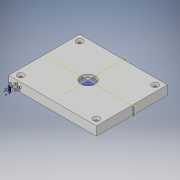
# Autodesk Inventor part: Masterboxtop
Saved by Autodesk Inventor 2019 (Build 230136000, 136)
## iProperties
Created: 2019-08-02
Part Number: Masterboxtop
Material: Generic
Document SubType Name: Modeling
Designer: Riley
Density: 1 g/cm^3
Appearance: Default
Author: Riley
Autodesk Inventor part; units mm, degrees
ref_plane "YZ Plane" through (0, 0, 0) normal (1, 0, 0) x (0, 1, 0)
ref_plane "XZ Plane" through (0, 0, 0) normal (0, 1, 0) x (-1, 0, 0)
ref_plane "XY Plane" through (0, 0, 0) normal (0, 0, 1) x (1, 0, 0)
sketch "Sketch1" plane through (0, 0, 0) normal (0, 1, 0) x (-1, 0, 0)
  line L0 (0, 0) -> (89.789, 0)
  line L1 (89.789, 0) -> (89.789, 71.3232)
  line L2 (89.789, 71.3232) -> (0, 71.3232)
  line L3 (0, 71.3232) -> (0, 0)
  line L4 (93.345, 74.8792) -> (-3.556, 74.8792)
  line L5 (-3.556, 74.8792) -> (-3.556, -3.556)
  line L6 (-3.556, -3.556) -> (93.345, -3.556)
  line L7 (93.345, -3.556) -> (93.345, 74.8792)
  dimension "d0" = 89.789
  dimension "d1" = 71.3232
  dimension "d2" = 3.556
  dimension "d3" = 3.556
  dimension "d4" = 3.556
  dimension "d5" = 3.556
  constraints: 16 end point, 4 parallel, 2 horizontal, 2 perpendicular
  measures "d0" distance of L2.end L1.end
  measures "d1" distance of L1.end L0.end
  measures "d2" distance between parallel lines of L4 L2
  measures "d3" distance between parallel lines of L7 L1
  measures "d4" distance between parallel lines of L6 L0
  measures "d5" distance between parallel lines of L5 L3
extrude "Extrusion1" add sketch "Sketch1" along normal blind 6.35
sketch "Sketch2" plane through (0, 6.35, 0) normal (0, 1, 0) x (1, 0, 0)
  line L0 (-93.345, 3.556) -> (3.556, 3.556)
  line L1 (3.556, 3.556) -> (3.556, -74.8792)
  line L2 (3.556, -74.8792) -> (-93.345, -74.8792)
  line L3 (-93.345, -74.8792) -> (-93.345, 3.556)
  point P0 (0, 0)
  dimension "d8" = 78.4352
  dimension "d9" = 96.901
  constraints: 8 end point, 2 parallel, 1 horizontal, 1 perpendicular
  measures "d8" distance between parallel lines of L2 L0
  measures "d9" distance between parallel lines of L1 L3
extrude "Extrusion2" add sketch "Sketch2" along normal blind 3.556
sketch "Sketch3" plane through (0, 9.906, 0) normal (0, 1, 0) x (1, 0, 0)
  circle A0 centre (-44.8945, -35.6616) radius 7.9883
  line L0 (-93.345, 3.556) -> (-93.345, -74.8792) projected
  line L1 (3.556, 3.556) -> (-93.345, 3.556) projected
  point P0 (0, 0)
  dimension "d12" = 48.4505
  dimension "d13" = 39.2176
  dimension "d14" = 15.9766
  constraints: 1 centre point
  measures "d12" distance from line of L0 A0.centre
  measures "d13" distance from line of L1 A0.centre
  measures "d14" diameter of A0
extrude "Extrusion3" cut sketch "Sketch3" against normal blind 3.556 and the other way blind 1.016
sketch "Sketch5" plane through (-93.345, 0, -3.556) normal (-1, 0, 0) x (0, 0, 1)
  line L0 (78.4352, 0) -> (0, 0) projected
  line L1 (78.4352, 0) -> (77.1652, 0)
  line L2 (77.1652, 0) -> (77.1652, -7.62)
  line L3 (77.1652, -7.62) -> (78.4352, -7.62)
  line L4 (78.4352, -7.62) -> (78.4352, 0)
  line L5 (77.1652, -7.62) -> (76.4032, -6.5318)
  line L6 (76.4032, -6.5318) -> (76.4032, -2.54)
  line L7 (76.4032, -2.54) -> (77.1652, -2.54)
  point P0 (3.556, 0)
  dimension "d19" = 1.27
  dimension "d20" = 7.62
  dimension "d21" = 35
  dimension "d22" = 5.08
  dimension "d23" = 0.762
  constraints: 14 end point, 2 parallel, 2 perpendicular, 1 horizontal, 1 point on line, 1 vertical
  measures "d19" distance between parallel lines of L2 L4
  measures "d20" distance between parallel lines of L0 L3
  measures "d21" angle of L5 L2
  measures "d22" distance between parallel lines of L3 L7
  measures "d23" distance between parallel lines of L2 L6
sketch "Sketch7" plane through (0, 9.906, 0) normal (0, 1, 0) x (1, 0, 0)
  circle A0 centre (-3.1305, -3.1305) radius 1.3525
  line L0 (0, 0) -> (0, -71.3232) projected
  line L1 (-89.789, 0) -> (0, 0) projected
  circle A1 centre (-3.1305, -3.1305) radius 3.1306
  dimension "d40" = 2.7051
  dimension "d41" = 6.2611
  constraints: 2 centre point, 2 tangent, 1 coincident
  measures "d40" diameter of A0
  measures "d41" diameter of A1
extrude "Extrusion6" cut sketch "Sketch7" along normal mid plane 25.4 contours A0
chamfer "Chamfer1" distance 1.905 angle 49 1 edges at (-4.4831, 9.906, 3.1305) measured on face at (-4.4831, 9.406, 3.1305)
ref_plane "Work Plane4" through (-44.8945, 0, -3.556) normal (-1, 0, 0) x (0, 0, 1)
ref_plane "Work Plane5" through (3.556, 0, 35.6616) normal (0, 0, -1) x (-1, 0, 0)
mirror "Mirror3" about plane through (3.556, 0, 35.6616) normal (0, 0, -1) of "Extrusion6", "Chamfer1"
mirror "Mirror4" about plane through (-44.8945, 0, -3.556) normal (-1, 0, 0) of "Extrusion6", "Chamfer1", "Mirror3"
equation "\"d3\" = d2"
equation "\"d4\" = d2"
equation "\"d5\" = d2"
equation "\"d8\" = d1 + 2 * d3"
equation "\"d9\" = d0 + 2 * d3"
equation "\"d10\" = d3"
equation "\"d12\" = 0.5 * d9"
equation "\"d13\" = 0.5 * d8"
equation "\"d15\" = d3"
equation "\"d47\" = -d2 - 0.5 * d0"
equation "\"d48\" = -0.5 * d1 - d2"
body "Solid1"
